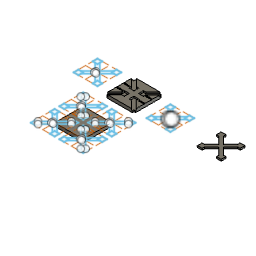
Bodenplatte_1 (Autodesk Fusion 360 design; units mm, degrees)
Autodesk Fusion 360 part; units mm, degrees
note: some values were not read from the file. Set by a fixed rule: which face or edge a step refers to.
(part 1 of 2)
sketch "Skizze1" plane through (0, 0, 0) normal (0, 1, 0) x (1, 0, 0)
  line L0 (-45, 40) -> (-45, -40)
  line L1 (-45, -40) -> (-40, -40)
  line L2 (-40, -40) -> (-40, -45)
  line L3 (-40, -45) -> (40, -45)
  line L4 (40, -45) -> (40, -40)
  line L5 (40, -40) -> (45, -40)
  line L6 (45, -40) -> (45, 40)
  line L7 (45, 40) -> (40, 40)
  line L8 (40, 40) -> (40, 45)
  line L9 (40, 45) -> (-40, 45)
  line L10 (-40, 45) -> (-40, 40)
  line L11 (-40, 40) -> (-45, 40)
  constraint vertical L0
  constraint perpendicular L0 L1
  constraint perpendicular L1 L2
  constraint perpendicular L2 L3
  constraint perpendicular L3 L4
  constraint perpendicular L4 L5
  constraint perpendicular L5 L6
  constraint perpendicular L6 L7
  constraint perpendicular L7 L8
  constraint perpendicular L8 L9
  constraint perpendicular L9 L10
  constraint perpendicular L0 L11
extrude "Extrusion1" add sketch "Skizze1" along normal blind 10 makes body 1
ref_plane "Arbeitsebene3" through (-45, 10, -40) normal (0, -1, 0) x (1, 0, 0)
sketch "Skizze5" plane through (0, 10, 0) normal (0, -1, 0) x (-1, 0, 0)
  line L0 (-7.5, -67.5) -> (-7.5, -82.5)
  line L1 (-22.5, -75) -> (-75, -22.5)
  line L2 (-75, -67.5) -> (-22.5, -15)
  line L3 (-67.5, -7.5) -> (-67.5, -22.5)
  line L4 (-22.5, -7.5) -> (-22.5, -22.5)
  line L5 (-7.5, -7.5) -> (-7.5, -82.5) construction
  line L6 (-15, -22.5) -> (-67.5, -75)
  line L7 (-67.5, -67.5) -> (-82.5, -67.5)
  line L8 (-7.5, -7.5) -> (-22.5, -7.5)
  line L9 (-22.5, -67.5) -> (-7.5, -67.5)
  line L10 (-7.5, -22.5) -> (-7.5, -7.5)
  line L11 (-7.5, -82.5) -> (-22.5, -82.5)
  line L12 (-22.5, -22.5) -> (-7.5, -22.5)
  line L13 (-45, -82.5) -> (-45, -7.5) construction
  line L14 (-22.5, -82.5) -> (-22.5, -67.5)
  line L15 (-67.5, -22.5) -> (-82.5, -22.5)
  line L16 (-82.5, -7.5) -> (-7.5, -7.5) construction
  line L17 (-82.5, -22.5) -> (-82.5, -7.5)
  line L18 (-7.5, -82.5) -> (-82.5, -82.5) construction
  line L19 (-67.5, -82.5) -> (-67.5, -67.5)
  line L20 (-82.5, -67.5) -> (-82.5, -82.5)
  line L21 (-82.5, -82.5) -> (-82.5, -7.5) construction
  line L22 (-82.5, -82.5) -> (-67.5, -82.5)
  line L23 (-82.5, -7.5) -> (-67.5, -7.5)
  line L24 (-15, -67.5) -> (-67.5, -15)
  line L25 (-7.5, -45) -> (-82.5, -45) construction
  line L26 (-7.4, -22.6) -> (-7.4, -7.4)
  line L27 (-7.4, -7.4) -> (-22.6, -7.4)
  line L28 (-22.6, -7.4) -> (-22.6, -22.6)
  line L29 (-22.6, -22.6) -> (-7.4, -22.6)
  line L30 (-75.0707, -67.4293) -> (-22.5707, -14.9293)
  line L31 (-14.9293, -22.5707) -> (-67.4293, -75.0707)
  point P0 (-40, -50)
  point P1 (-45, -50)
  point P2 (-40, -45)
  dimension "d20" = 75
  dimension "d21" = 75
  dimension "d22" = 0.1
  dimension "d23" = -0.1
  dimension "d24" = -0.1
  constraint horizontal L18
  constraint vertical L21
  constraint horizontal L16
  constraint vertical L5
  constraint horizontal L11
  constraint vertical L14
  constraint horizontal L9
  constraint vertical L0
  constraint horizontal L22
  constraint vertical L19
  constraint horizontal L7
  constraint vertical L20
  constraint horizontal L8
  constraint vertical L4
  constraint horizontal L12
  constraint vertical L10
  constraint horizontal L23
  constraint vertical L3
  constraint horizontal L15
  constraint vertical L17
  constraint midpoint L6.start L12
  constraint midpoint L6.end L19
  constraint midpoint L2.start L7
  constraint midpoint L2.end L4
  constraint midpoint L24.start L9
  constraint midpoint L24.end L3
  constraint midpoint L1.start L14
  constraint midpoint L1.end L15
  constraint midpoint L13.start L18
  constraint midpoint L13.end L16
  constraint midpoint L25.start L5
  constraint midpoint L25.end L21
  measures "d20" distance of L0.end L18.end
  measures "d21" distance of L5.start L0.end
extrude "Extrusion2" cut sketch "Skizze5" along normal blind 5 contours L1 L6 L24 L31 | L6 L24 L29 L31 | L2 L6 L24 L28 L29 | L1 L2 L6 L24 | L2 L4 L6 L8 L10 L12 L26 L27 L28 L29 | L2 L4 L6 L12 L28 L29 | L2 L24 L28 L30 | L1 L2 L24 L30 | L4 L8 L10 L12 bodies 1
ref_plane "Arbeitsebene4" through (-45, 10, -40) normal (0, -1, 0) x (1, 0, 0)
sketch "Skizze6" plane through (0, 10, 0) normal (0, -1, 0) x (-1, 0, 0)
  line L0 (-26.2733, -14.8317) -> (-41.3593, -14.8317) construction
  line L1 (-41.3593, -14.8317) -> (-41.3593, -8.56) construction
  line L2 (-41.3593, -8.56) -> (-26.2733, -8.56) construction
  line L3 (-26.2733, -8.56) -> (-26.2733, -14.8317) construction
  dimension "d27" = 4
  text T0 "0,1mm" font "Arial" height 4 align left top in box 15.086 x 6.2717 at (-26.2733, -14.8317) x (-1, 0) y (0, 1) spacing 1 kerned
extrude "Extrusion3" cut sketch "Skizze6" along normal blind 1 text T0 bodies 1
ref_plane "Arbeitsebene5" through (-45, 10, -40) normal (0, -1, 0) x (1, 0, 0)
sketch "Skizze7" plane through (0, 10, 0) normal (0, -1, 0) x (-1, 0, 0)
  line L0 (82.5, -67.5) -> (82.5, -82.5)
  line L1 (67.5, -75) -> (15, -22.5)
  line L2 (15, -67.5) -> (67.5, -15)
  line L3 (22.5, -7.5) -> (22.5, -22.5)
  line L4 (67.5, -7.5) -> (67.5, -22.5)
  line L5 (82.5, -7.5) -> (82.5, -82.5) construction
  line L6 (75, -22.5) -> (22.5, -75)
  line L7 (22.5, -67.5) -> (7.5, -67.5)
  line L8 (82.5, -7.5) -> (67.5, -7.5)
  line L9 (67.5, -67.5) -> (82.5, -67.5)
  line L10 (82.5, -22.5) -> (82.5, -7.5)
  line L11 (82.5, -82.5) -> (67.5, -82.5)
  line L12 (67.5, -22.5) -> (82.5, -22.5)
  line L13 (45, -82.5) -> (45, -7.5) construction
  line L14 (67.5, -82.5) -> (67.5, -67.5)
  line L15 (22.5, -22.5) -> (7.5, -22.5)
  line L16 (7.5, -7.5) -> (82.5, -7.5) construction
  line L17 (7.5, -22.5) -> (7.5, -7.5)
  line L18 (82.5, -82.5) -> (7.5, -82.5) construction
  line L19 (22.5, -82.5) -> (22.5, -67.5)
  line L20 (7.5, -67.5) -> (7.5, -82.5)
  line L21 (7.5, -82.5) -> (7.5, -7.5) construction
  line L22 (7.5, -82.5) -> (22.5, -82.5)
  line L23 (7.5, -7.5) -> (22.5, -7.5)
  line L24 (75, -67.5) -> (22.5, -15)
  line L25 (82.5, -45) -> (7.5, -45) construction
  line L26 (75.1061, -67.3939) -> (22.6061, -14.8939)
  line L27 (67.3939, -75.1061) -> (14.8939, -22.6061)
  line L28 (7.35, -7.35) -> (22.65, -7.35)
  line L29 (22.65, -7.35) -> (22.65, -22.65)
  line L30 (22.65, -22.65) -> (7.35, -22.65)
  line L31 (7.35, -22.65) -> (7.35, -7.35)
  point P0 (50, -50)
  point P1 (45, -50)
  point P2 (50, -45)
  dimension "d30" = 75
  dimension "d31" = 75
  dimension "d32" = 0.15
  dimension "d33" = -0.15
  dimension "d34" = -0.15
  constraint horizontal L18
  constraint vertical L21
  constraint horizontal L16
  constraint vertical L5
  constraint horizontal L11
  constraint vertical L14
  constraint horizontal L9
  constraint vertical L0
  constraint horizontal L22
  constraint vertical L19
  constraint horizontal L7
  constraint vertical L20
  constraint horizontal L8
  constraint vertical L4
  constraint horizontal L12
  constraint vertical L10
  constraint horizontal L23
  constraint vertical L3
  constraint horizontal L15
  constraint vertical L17
  constraint midpoint L6.start L12
  constraint midpoint L6.end L19
  constraint midpoint L2.start L7
  constraint midpoint L2.end L4
  constraint midpoint L24.start L9
  constraint midpoint L24.end L3
  constraint midpoint L1.start L14
  constraint midpoint L1.end L15
  constraint midpoint L13.start L18
  constraint midpoint L13.end L16
  constraint midpoint L25.start L5
  constraint midpoint L25.end L21
  measures "d30" distance of L0.end L18.end
  measures "d31" distance of L5.start L0.end
extrude "Extrusion4" cut sketch "Skizze7" along normal blind 5 contours L2 L6 L24 L26 | L1 L2 L6 L24 | L1 L2 L6 L27 | L2 L24 L26 L29 | L1 L2 L24 L29 L30 | L1 L2 L27 L30 | L1 L3 L15 L24 L29 L30 | L1 L3 L15 L17 L23 L24 L28 L29 L30 L31 | L3 L15 L17 L23 bodies 1
ref_plane "Arbeitsebene6" through (-45, 10, -40) normal (0, -1, 0) x (1, 0, 0)
sketch "Skizze8" plane through (0, 10, 0) normal (0, -1, 0) x (-1, 0, 0)
  line L0 (43.5802, -15.8742) -> (43.5801, -15.8742) construction
  line L1 (43.5801, -15.8742) -> (43.7283, -9.6192) construction
  line L2 (43.7283, -9.6192) -> (43.7284, -9.6192) construction
  line L3 (43.7284, -9.6192) -> (43.5802, -15.8742) construction
  line L4 (82.5, 22.5) -> (82.5, 7.5)
  line L5 (67.5, 15) -> (15, 67.5)
  line L6 (15, 22.5) -> (67.5, 75)
  line L7 (22.5, 82.5) -> (22.5, 67.5)
  line L8 (67.5, 82.5) -> (67.5, 67.5)
  line L9 (82.5, 82.5) -> (82.5, 7.5) construction
  line L10 (75, 67.5) -> (22.5, 15)
  line L11 (22.5, 22.5) -> (7.5, 22.5)
  line L12 (82.5, 82.5) -> (67.5, 82.5)
  line L13 (67.5, 22.5) -> (82.5, 22.5)
  line L14 (82.5, 67.5) -> (82.5, 82.5)
  line L15 (82.5, 7.5) -> (67.5, 7.5)
  line L16 (67.5, 67.5) -> (82.5, 67.5)
  line L17 (45, 7.5) -> (45, 82.5) construction
  line L18 (67.5, 7.5) -> (67.5, 22.5)
  line L19 (22.5, 67.5) -> (7.5, 67.5)
  line L20 (7.5, 82.5) -> (82.5, 82.5) construction
  line L21 (7.5, 67.5) -> (7.5, 82.5)
  line L22 (82.5, 7.5) -> (7.5, 7.5) construction
  line L23 (22.5, 7.5) -> (22.5, 22.5)
  line L24 (7.5, 22.5) -> (7.5, 7.5)
  line L25 (7.5, 7.5) -> (7.5, 82.5) construction
  line L26 (7.5, 7.5) -> (22.5, 7.5)
  line L27 (7.5, 82.5) -> (22.5, 82.5)
  line L28 (75, 22.5) -> (22.5, 75)
  line L29 (82.5, 45) -> (7.5, 45) construction
  line L30 (14.8586, 22.6414) -> (67.3586, 75.1414)
  line L31 (75.1414, 67.3586) -> (22.6414, 14.8586)
  line L32 (22.7, 22.7) -> (7.3, 22.7)
  line L33 (7.3, 22.7) -> (7.3, 7.3)
  line L34 (7.3, 7.3) -> (22.7, 7.3)
  line L35 (22.7, 7.3) -> (22.7, 22.7)
  line L36 (-7.5, 22.5) -> (-7.5, 7.5)
  line L37 (-22.5, 15) -> (-75, 67.5)
  line L38 (-75, 22.5) -> (-22.5, 75)
  line L39 (-67.5, 82.5) -> (-67.5, 67.5)
  line L40 (-22.5, 82.5) -> (-22.5, 67.5)
  line L41 (-7.5, 82.5) -> (-7.5, 7.5) construction
  line L42 (-15, 67.5) -> (-67.5, 15)
  line L43 (-67.5, 22.5) -> (-82.5, 22.5)
  line L44 (-7.5, 82.5) -> (-22.5, 82.5)
  line L45 (-22.5, 22.5) -> (-7.5, 22.5)
  line L46 (-7.5, 67.5) -> (-7.5, 82.5)
  line L47 (-7.5, 7.5) -> (-22.5, 7.5)
  line L48 (-22.5, 67.5) -> (-7.5, 67.5)
  line L49 (-45, 7.5) -> (-45, 82.5) construction
  line L50 (-22.5, 7.5) -> (-22.5, 22.5)
  line L51 (-67.5, 67.5) -> (-82.5, 67.5)
  line L52 (-82.5, 82.5) -> (-7.5, 82.5) construction
  line L53 (-82.5, 67.5) -> (-82.5, 82.5)
  line L54 (-7.5, 7.5) -> (-82.5, 7.5) construction
  line L55 (-67.5, 7.5) -> (-67.5, 22.5)
  line L56 (-82.5, 22.5) -> (-82.5, 7.5)
  line L57 (-82.5, 7.5) -> (-82.5, 82.5) construction
  line L58 (-82.5, 7.5) -> (-67.5, 7.5)
  line L59 (-82.5, 82.5) -> (-67.5, 82.5)
  line L60 (-15, 22.5) -> (-67.5, 75)
  line L61 (-7.5, 45) -> (-82.5, 45) construction
  line L62 (-22.6768, 14.8232) -> (-75.1768, 67.3232)
  line L63 (-14.8232, 22.6768) -> (-67.3232, 75.1768)
  line L64 (-7.25, 7.25) -> (-22.75, 7.25)
  line L65 (-22.75, 7.25) -> (-22.75, 22.75)
  line L66 (-22.75, 22.75) -> (-7.25, 22.75)
  line L67 (-7.25, 22.75) -> (-7.25, 7.25)
  line L68 (43.7513, 9) -> (26, 9) construction
  line L69 (26, 9) -> (26, 17.5106) construction
  line L70 (26, 17.5106) -> (43.7513, 17.5106) construction
  line L71 (43.7513, 17.5106) -> (43.7513, 9) construction
  line L72 (-24.3671, 8.4428) -> (-42.7802, 8.4428) construction
  line L73 (-42.7802, 8.4428) -> (-42.7802, 14.5497) construction
  line L74 (-42.7802, 14.5497) -> (-24.3671, 14.5497) construction
  line L75 (-24.3671, 14.5497) -> (-24.3671, 8.4428) construction
  point P0 (50, 40)
  point P1 (45, 40)
  point P2 (50, 45)
  point P3 (-40, 40)
  point P4 (-45, 40)
  point P5 (-40, 45)
  dimension "d37" = 4
  dimension "d38" = 75
  dimension "d39" = 75
  dimension "d40" = -0.2
  dimension "d41" = -0.2
  dimension "d42" = 0.2
  dimension "d43" = 75
  dimension "d44" = 75
  dimension "d45" = -0.25
  dimension "d46" = 0.25
  dimension "d47" = -0.25
  dimension "d48" = 4
  dimension "d49" = 4
  constraint horizontal L22
  constraint vertical L25
  constraint horizontal L20
  constraint vertical L9
  constraint horizontal L15
  constraint vertical L18
  constraint horizontal L13
  constraint vertical L4
  constraint horizontal L26
  constraint vertical L23
  constraint horizontal L11
  constraint vertical L24
  constraint horizontal L12
  constraint vertical L8
  constraint horizontal L16
  constraint vertical L14
  constraint horizontal L27
  constraint vertical L7
  constraint horizontal L19
  constraint vertical L21
  constraint midpoint L10.start L16
  constraint midpoint L10.end L23
  constraint midpoint L6.start L11
  constraint midpoint L6.end L8
  constraint midpoint L28.start L13
  constraint midpoint L28.end L7
  constraint midpoint L5.start L18
  constraint midpoint L5.end L19
  constraint midpoint L17.start L22
  constraint midpoint L17.end L20
  constraint midpoint L29.start L9
  constraint midpoint L29.end L25
  constraint horizontal L54
  constraint vertical L57
  constraint horizontal L52
  constraint vertical L41
  constraint horizontal L47
  constraint vertical L50
  constraint horizontal L45
  constraint vertical L36
  constraint horizontal L58
  constraint vertical L55
  constraint horizontal L43
  constraint vertical L56
  constraint horizontal L44
  constraint vertical L40
  constraint horizontal L48
  constraint vertical L46
  constraint horizontal L59
  constraint vertical L39
  constraint horizontal L51
  constraint vertical L53
  constraint midpoint L42.start L48
  constraint midpoint L42.end L55
  constraint midpoint L38.start L43
  constraint midpoint L38.end L40
  constraint midpoint L60.start L45
  constraint midpoint L60.end L39
  constraint midpoint L37.start L50
  constraint midpoint L37.end L51
  constraint midpoint L49.start L54
  constraint midpoint L49.end L52
  constraint midpoint L61.start L41
  constraint midpoint L61.end L57
  measures "d38" distance of L4.end L22.end
  measures "d39" distance of L9.start L4.end
  measures "d43" distance of L36.end L54.end
  measures "d44" distance of L41.start L36.end
sketch "Skizze9" plane through (0, 0, 0) normal (0, 0, 1) x (1, 0, 0)
extrude "Extrusion5" cut sketch "Skizze8" along normal blind 5 contours L5 L10 L28 L31 | L5 L6 L10 L28 | L5 L10 L31 L35 | L5 L6 L10 L32 L35 | L5 L6 L28 L30 | L6 L10 L11 L23 L24 L26 L32 L33 L34 L35 | L5 L6 L30 L32 | L6 L10 L11 L23 L32 L35 | L11 L23 L24 L26 | L36 L37 L45 L47 L50 L60 L64 L65 L66 L67 | L36 L45 L47 L50 | L37 L45 L50 L60 L65 L66 | L37 L42 L60 L65 L66 | L42 L60 L63 L66 | L38 L42 L60 L63 | L37 L38 L42 L60 | L37 L42 L62 L65 | L37 L38 L42 L62 bodies 1
ref_plane "Arbeitsebene7" through (-45, 10, -37.2172) normal (0, -1, 0) x (1, 0, 0)
sketch "Skizze10" plane through (0, 10, 0) normal (0, -1, 0) x (-1, 0, 0)
  line L0 (44, -14) -> (25, -14) construction
  line L1 (25, -14) -> (25, -7) construction
  line L2 (25, -7) -> (44, -7) construction
  line L3 (44, -7) -> (44, -14) construction
  line L4 (43, 8.2933) -> (24.4104, 8.2933) construction
  line L5 (24.4104, 8.2933) -> (24.4104, 15) construction
  line L6 (24.4104, 15) -> (43, 15) construction
  line L7 (43, 15) -> (43, 8.2933) construction
  line L8 (-24, 9) -> (-42, 9) construction
  line L9 (-42, 9) -> (-42, 15) construction
  line L10 (-42, 15) -> (-24, 15) construction
  line L11 (-24, 15) -> (-24, 9) construction
  dimension "d52" = 4
  dimension "d53" = 4
  dimension "d54" = 4
  text T0 "0,15mm" font "Arial" height 4 align left top in box 19 x 7 at (44, -14) x (-1, 0) y (0, 1) spacing 1 kerned
  text T1 "0,2mm" font "Arial" height 4 align left top in box 18.5896 x 6.7067 at (43, 8.2933) x (-1, 0) y (0, 1) spacing 1 kerned
  text T2 "0,25mm" font "Arial" height 4 align left top in box 18 x 6 at (-24, 9) x (-1, 0) y (0, 1) spacing 1 kerned
extrude "Extrusion6" cut sketch "Skizze10" along normal blind 1 text T2 T1 T0 bodies 1
sketch "Skizze11" plane through (0, 0, 0) normal (0, 0, 1) x (1, 0, 0)
sketch "Skizze12" plane through (0, 0, 0) normal (0, 1, 0) x (1, 0, 0)
  line L0 (152.5, -22.5) -> (152.5, -37.5)
  line L1 (137.5, -30) -> (85, 22.5)
  line L2 (85, -22.5) -> (137.5, 30)
  line L3 (92.5, 37.5) -> (92.5, 22.5)
  line L4 (137.5, 37.5) -> (137.5, 22.5)
  line L5 (152.5, 37.5) -> (152.5, -37.5) construction
  line L6 (145, 22.5) -> (92.5, -30)
  line L7 (92.5, -22.5) -> (77.5, -22.5)
  line L8 (152.5, 37.5) -> (137.5, 37.5)
  line L9 (137.5, -22.5) -> (152.5, -22.5)
  line L10 (152.5, 22.5) -> (152.5, 37.5)
  line L11 (152.5, -37.5) -> (137.5, -37.5)
  line L12 (137.5, 22.5) -> (152.5, 22.5)
  line L13 (115, -37.5) -> (115, 37.5) construction
  line L14 (137.5, -37.5) -> (137.5, -22.5)
  line L15 (92.5, 22.5) -> (77.5, 22.5)
  line L16 (77.5, 37.5) -> (152.5, 37.5) construction
  line L17 (77.5, 22.5) -> (77.5, 37.5)
  line L18 (152.5, -37.5) -> (77.5, -37.5) construction
  line L19 (92.5, -37.5) -> (92.5, -22.5)
  line L20 (77.5, -22.5) -> (77.5, -37.5)
  line L21 (77.5, -37.5) -> (77.5, 37.5) construction
  line L22 (77.5, -37.5) -> (92.5, -37.5)
  line L23 (77.5, 37.5) -> (92.5, 37.5)
  line L24 (145, -22.5) -> (92.5, 30)
  line L25 (152.5, 0) -> (77.5, 0) construction
  point P0 (120, -5)
  point P1 (115, -5)
  point P2 (120, 0)
  dimension "d57" = 75
  dimension "d58" = 75
  constraint horizontal L18
  constraint vertical L21
  constraint horizontal L16
  constraint vertical L5
  constraint horizontal L11
  constraint vertical L14
  constraint horizontal L9
  constraint vertical L0
  constraint horizontal L22
  constraint vertical L19
  constraint horizontal L7
  constraint vertical L20
  constraint horizontal L8
  constraint vertical L4
  constraint horizontal L12
  constraint vertical L10
  constraint horizontal L23
  constraint vertical L3
  constraint horizontal L15
  constraint vertical L17
  constraint midpoint L6.start L12
  constraint midpoint L6.end L19
  constraint midpoint L2.start L7
  constraint midpoint L2.end L4
  constraint midpoint L24.start L9
  constraint midpoint L24.end L3
  constraint midpoint L1.start L14
  constraint midpoint L1.end L15
  constraint midpoint L13.start L18
  constraint midpoint L13.end L16
  constraint midpoint L25.start L5
  constraint midpoint L25.end L21
  measures "d57" distance of L0.end L18.end
  measures "d58" distance of L5.start L0.end
extrude "Extrusion7" add sketch "Skizze12" along normal blind 5 separate body makes body 2
copy_body "Körper kopieren/einfügen1" bodies 2 makes body 3
move_body "Verschieben2" bodies 3 to x (1, 0, 0) y (0, 1, 0) z (0, 0, 1) at (160, 0, 0)
copy_body "Körper kopieren/einfügen2" bodies 1 makes body 4
move_body "Verschieben3" bodies 4 to x (1, 0, 0) y (0, 1, 0) z (0, 0, 1) at (0, 0, 160)
extrude "Extrusion8" add 4 faces at (25.8821, 5, 134.1179) (-25.8724, 5, 134.1276) (-25.8626, 5, 185.8626) (25.8529, 5, 185.8529) along direction (0, 1, 0) blind 5 on bodies 4 bodies 4
delete_face "Fläche löschen1" 236 faces at (-29.9479, 9.5, 147.3795) (-40.0682, 9.3333, 170.6271) (-24.5694, 9.6667, 171) (-30.9386, 9.6667, 171) (-31.697, 9.5, 168.4677) (-34.6562, 9.6667, 146.2378) (-40.5885, 9.5, 148.2966) (-42.7174, 9.5, 148.4385) (-41.5585, 9.5, 149.059) (-41.8758, 9.5, 149.0506) (-42.4956, 9.5, 147.3048) (-42.1855, 9.5, 148.4319) (-41.206, 9.5, 148.4309) (-41.0614, 9.5, 148.1749) (-40.8959, 9.5, 146.7492) (-42.3137, 9.5, 145.8483) (-42.6525, 9, 147.3777) (-26.6771, 9.6667, 149) (-35.0941, 9.6667, 167.0546) (-30.162, 9.5, 168.4713) (-31.1692, 9.3333, 147.6739) (-39.0716, 9.5, 149.0942) (-39.4515, 9.5, 149.7541) (-39.5694, 9.3333, 149.7212) (-26.1201, 9.6667, 169.8777) (-34.0396, 9.5, 170.7219) (-41.5885, 9.5, 170.2966) (-43.7174, 9.5, 170.4385) (-30.2769, 9, 147.533) (-42.5585, 9.5, 171.059) (-37.1921, 9.5, 147.3665) (-42.8758, 9.5, 171.0506) (-37.1319, 9.5, 145.3985) (-43.4956, 9.5, 169.3048) (-43.1855, 9.5, 170.4319) (-37.7964, 9.5, 146.0767) (-29.0614, 9.3333, 169.6739) (-33.3766, 9.5, 147.0199) (-29.2242, 9.6667, 171) (-34.1096, 9.5, 169.5582) (-33.3738, 9.3333, 148.3724) (-26.075, 9.5, 168.3987) (-40.0716, 9.5, 171.0942) (-35.4361, 9.6667, 167.8822) (-32.8376, 9.5, 146.3987) (-24.895, 9.3333, 170.3915) (-35.4598, 9.5, 168.5269) (-40.4515, 9.5, 171.7541) (-32.9926, 9.5, 146.4694) (-24.8954, 9.5, 169.0897) (-27.0032, 9.5, 147.0897) (-33.6782, 9.5, 146.0414) (-40.5694, 9.3333, 171.7212) (-34.6573, 9.5, 168.3643) (-25.0779, 9.5, 168.5699) (-27.1856, 9.5, 146.5699) (-33.5948, 9.5, 169.4652) (-40.442, 9.6667, 171) (-31.266, 9.3333, 170.3724) (-25.357, 9.5, 168.4657) (-27.4647, 9.5, 146.4657) (-29.8401, 9.5, 146.8259) (-30.1132, 9.6667, 149) (-42.206, 9.5, 170.4309) (-32.1196, 9.5, 146.4657) (-31.8405, 9.5, 146.5699) (-26.5206, 9.5, 146.8624) (-35.8372, 9.3333, 169.1492) (-31.658, 9.5, 147.0897) (-31.6576, 9.3333, 148.3915) (-26.5143, 9.3333, 147.6739) (-36.0155, 9.6667, 168.4243) (-31.332, 9.6667, 149) (-30.0118, 9.5, 168.4657) (-29.5498, 9.3333, 170.3915) (-33.0464, 9.6667, 149) (-34.8357, 9.5, 168.7917) (-29.5503, 9.5, 169.0897) (-41.8959, 9.5, 168.7492) (-43.3137, 9.5, 167.8483) (-34.3645, 9.5, 146.2132) (-40.6126, 9.5, 171.5561) (-31.9326, 9.5, 146.045) (-33.5936, 9.5, 169.8169) (-40.3483, 9, 170.6271) (-25.5071, 9.5, 168.4713) (-36.2033, 9.5, 170.11) (-27.6149, 9.5, 146.4713) (-38.0896, 9.5, 148.2126) (-37.5053, 9.5, 147.6264) (-42.2066, 9.5, 167.6217) (-39.4411, 9.6667, 148.4407) (-42.4342, 10, 168.7024) (-39.0682, 9.3333, 148.6271) (-43.1684, 9.5, 167.5944) (-40.3533, 9.5, 171.074) (-33.8048, 9.5, 146.4677) (-29.0676, 9.5, 168.8624) (-37.1865, 9.5, 144.9942) (-37.2938, 9, 148.8427) (-37.0677, 9.5, 147.8608) (-37.5523, 9.5, 148.3053) (-43.6525, 9, 169.3777) (-39.6276, 9.3333, 148.8136) (-28.0055, 9.6667, 171) (-32.495, 9.5, 169.3795) (-42.8323, 9.5, 166.9929) (-38.4011, 9.5, 148.9416) (-28.1692, 9, 169.533) (-32.4966, 9.6667, 169.9977) (-42.5937, 9.5, 166.9888) (-25.17, 9.5, 168.045) (-31.1754, 9.5, 146.8624) (-30.77, 9.5, 169.1837) (-27.0027, 9.3333, 148.3915) (-34.3001, 9.6667, 167.5239) (-32.2567, 9.5, 168.2132) (-37.4898, 9.3333, 168.3224) (-29.0234, 9.5, 146.0414) (-27.6018, 9.5, 168.2132) (-36.2783, 9.5, 145.9902) (-28.3377, 9.5, 146.4694) (-27.1075, 9.5, 168.0423) (-36.4323, 9.5, 146.5757) (-31.7624, 9.5, 168.0423) (-37.6535, 9, 168.618) (-35.7585, 9.6667, 148.6853) (-34.4331, 9.5, 170.4737) (-31.5705, 9.5, 168.0414) (-34.6044, 9.6667, 147.9977) (-34.1102, 9.5, 169.8244) (-30.8848, 9.5, 168.4694) (-34.6028, 9.5, 147.3795) (-38.1506, 9.5, 167.4315) (-26.9156, 9.5, 168.0414) (-30.7298, 9.5, 168.3987) (-28.1828, 9.5, 146.3987) (-34.9318, 9, 147.533) (-26.23, 9.5, 168.4694) (-37.7008, 9.6667, 166.9836) (-34.7681, 9.6667, 149) (-33.8702, 9.5, 146.0423) (-31.2689, 9.5, 169.0199) (-41.786, 9.5, 167.4112) (-29.15, 9.5, 146.4677) (-33.7681, 9.3333, 167.211) (-41.2066, 9.5, 145.6217) (-41.4342, 10, 146.7024) (-28.2229, 9.5, 147.1837) (-26.2838, 9.6667, 171) (-43.9961, 9.5, 168.8128) (-35.0955, 9.6667, 148.0341) (-28.2278, 9.6667, 147.8777) (-32.3872, 9.5, 168.8259) (-26.6112, 9.3333, 170.3724) (-32.6603, 9.6667, 171) (-26.614, 9.5, 169.0199) (-43.8014, 9.5, 167.7526) (-28.3915, 9.6667, 149) (-35.1168, 9.5, 171.0563) (-27.0422, 9.5, 168.4677) (-28.719, 9.3333, 148.3724) (-32.824, 9, 169.533) (-27.1918, 9.5, 168.4675) (-27.7324, 9.5, 168.8259) (-36.6398, 9.6667, 149) (-33.9544, 9.5, 146.4675) (-29.8248, 9.5, 168.045) (-37.9732, 9.6667, 146.1751) (-42.0614, 9.5, 170.1749) (-28.7218, 9.5, 147.0199) (-30.7749, 9.6667, 169.8777) (-34.495, 9.5, 146.8259) (-38.2827, 9.5, 145.968) (-32.8827, 9.6667, 147.8777) (-35.0313, 9.5, 168.7864) (-32.8778, 9.5, 147.1837) (-40.6276, 9.3333, 170.8136) (-24.4128, 9.5, 168.8624) (-35.4429, 9.5, 168.9279) (-27.2778, 9.5, 146.045) (-32.2698, 9.5, 146.4713) (-40.4411, 9.6667, 170.4407) (-24.4065, 9.3333, 169.6739) (-29.7327, 9.5, 168.5699) (-42.1684, 9.5, 145.5944) (-36.06, 9.6667, 169.9377) (-39.442, 9.6667, 149) (-39.3483, 9, 148.6271) (-39.6126, 9.5, 149.5561) (-39.3533, 9.5, 149.074) (-42.9961, 9.5, 146.8128) (-42.8014, 9.5, 145.7526) (-41.8323, 9.5, 144.9929) (-41.5937, 9.5, 144.9888) (-40.786, 9.5, 145.4112) (-40.5133, 9.5, 145.9722) (-40.3937, 9.5, 146.8488) (-40.3955, 9.5, 147.2404) (-26.1151, 9.5, 169.1837) (-34.9632, 9, 167.211) (-41.5133, 9.5, 167.9722) (-41.3937, 9.5, 168.8488) (-29.2996, 9.5, 146.4675) (-41.3955, 9.5, 169.2404) (-31.8467, 9.5, 168.4675) (-34.9491, 9.6667, 146.1023) (-27.8401, 9.5, 169.3795) (-38.3577, 9.5, 168.1546) (-28.1864, 9.6667, 168.1023) (-30.0014, 9.6667, 146.2378) (-35.693, 9.5, 170.0227) (-32.8413, 9.6667, 168.1023) (-38.5362, 9.5, 168.26) (-32.9877, 9.6667, 170.0341) (-37.6535, 9.6667, 171) (-37.0664, 9.6667, 148.528) (-35.7793, 9.5, 145.9441) (-29.2153, 9.5, 146.0423) (-36.8336, 9.5, 144.9953) (-38.8318, 9.5, 167.9204) (-35.0407, 9.5, 170.656) (-27.8936, 9.6667, 168.2378) (-36.1197, 9.5, 146.9734) (-30.2942, 9.6667, 146.1023) (-35.834, 9.5, 146.4889) (-29.9495, 9.6667, 147.9977) (-27.8417, 9.6667, 169.9977) (-36.7918, 9.5, 147.6278) (-30.4407, 9.6667, 148.0341) (-29.7096, 9.5, 146.2132) (-37.9809, 9.3333, 169.9568) (-28.3329, 9.6667, 170.0341) (-38.9632, 9.6667, 168.3042) (-32.5484, 9.6667, 168.2378) (-36.9172, 9.5, 145.3982) on bodies 4
extrude "Extrusion9" add 6 faces at (24.3475, 9, 147.3777) (27.6517, 9, 148.6271) (29.7062, 9, 148.8427) (33.0368, 9, 145.211) (35.176, 9, 147.533) (39.8308, 9, 147.533) along direction (0, 1, 0) blind 1 on bodies 4 bodies 4
extrude "Extrusion10" add 5 faces at (26.6208, 9, 170.9377) (29.925, 9, 172.1871) (32.6198, 9, 170.178) (34.3415, 9, 171.093) (38.9964, 9, 171.093) along direction (0, 1, 0) blind 1 on bodies 4 bodies 4
ref_plane "Arbeitsebene8" through (-45, 10, 120) normal (0, -1, 0) x (1, 0, 0)
sketch "Skizze13" plane through (0, 10, 0) normal (0, -1, 0) x (-1, 0, 0)
  line L0 (77.5, -37.5) -> (92.5, -37.5)
  line L1 (152.5, -37.5) -> (77.5, -37.5) construction
  line L2 (77.5, 22.5) -> (77.5, 37.5)
  line L3 (137.5, -22.5) -> (152.5, -22.5)
  line L4 (152.5, -22.5) -> (152.5, -37.5)
  line L5 (152.5, 0) -> (77.5, 0) construction
  line L6 (145, -22.5) -> (92.5, 30)
  line L7 (92.5, -37.5) -> (92.5, -22.5)
  line L8 (137.5, 37.5) -> (137.5, 22.5)
  line L9 (137.5, 22.5) -> (152.5, 22.5)
  line L10 (77.5, 37.5) -> (152.5, 37.5) construction
  line L11 (152.5, 22.5) -> (152.5, 37.5)
  line L12 (115, -37.5) -> (115, 37.5) construction
  line L13 (77.5, -37.5) -> (77.5, 37.5) construction
  line L14 (145, 22.5) -> (92.5, -30)
  line L15 (137.5, -30) -> (85, 22.5)
  line L16 (85, -22.5) -> (137.5, 30)
  line L17 (152.5, 37.5) -> (152.5, -37.5) construction
  line L18 (152.5, 37.5) -> (137.5, 37.5)
  line L19 (92.5, 22.5) -> (77.5, 22.5)
  line L20 (77.5, -22.5) -> (77.5, -37.5)
  line L21 (152.5, -37.5) -> (137.5, -37.5)
  line L22 (92.5, -22.5) -> (77.5, -22.5)
  line L23 (77.5, 37.5) -> (92.5, 37.5)
  line L24 (92.5, 37.5) -> (92.5, 22.5)
  line L25 (137.5, -37.5) -> (137.5, -22.5)
  line L26 (-82.5, -242.5) -> (-67.5, -242.5)
  line L27 (-7.5, -242.5) -> (-82.5, -242.5) construction
  line L28 (-82.5, -182.5) -> (-82.5, -167.5)
  line L29 (-22.5, -227.5) -> (-7.5, -227.5)
  line L30 (-7.5, -227.5) -> (-7.5, -242.5)
  line L31 (-7.5, -205) -> (-82.5, -205) construction
  line L32 (-15, -227.5) -> (-67.5, -175)
  line L33 (-67.5, -242.5) -> (-67.5, -227.5)
  line L34 (-22.5, -167.5) -> (-22.5, -182.5)
  line L35 (-22.5, -182.5) -> (-7.5, -182.5)
  line L36 (-82.5, -167.5) -> (-7.5, -167.5) construction
  line L37 (-7.5, -182.5) -> (-7.5, -167.5)
  line L38 (-45, -242.5) -> (-45, -167.5) construction
  line L39 (-82.5, -242.5) -> (-82.5, -167.5) construction
  line L40 (-15, -182.5) -> (-67.5, -235)
  line L41 (-22.5, -235) -> (-75, -182.5)
  line L42 (-75, -227.5) -> (-22.5, -175)
  line L43 (-7.5, -167.5) -> (-7.5, -242.5) construction
  line L44 (-7.5, -167.5) -> (-22.5, -167.5)
  line L45 (-67.5, -182.5) -> (-82.5, -182.5)
  line L46 (-82.5, -227.5) -> (-82.5, -242.5)
  line L47 (-7.5, -242.5) -> (-22.5, -242.5)
  line L48 (-67.5, -227.5) -> (-82.5, -227.5)
  line L49 (-82.5, -167.5) -> (-67.5, -167.5)
  line L50 (-67.5, -167.5) -> (-67.5, -182.5)
  line L51 (-22.5, -242.5) -> (-22.5, -227.5)
  line L52 (7.5, -242.5) -> (22.5, -242.5)
  line L53 (82.5, -242.5) -> (7.5, -242.5) construction
  line L54 (7.5, -182.5) -> (7.5, -167.5)
  line L55 (67.5, -227.5) -> (82.5, -227.5)
  line L56 (82.5, -227.5) -> (82.5, -242.5)
  line L57 (82.5, -205) -> (7.5, -205) construction
  line L58 (75, -227.5) -> (22.5, -175)
  line L59 (22.5, -242.5) -> (22.5, -227.5)
  line L60 (67.5, -167.5) -> (67.5, -182.5)
  line L61 (67.5, -182.5) -> (82.5, -182.5)
  line L62 (7.5, -167.5) -> (82.5, -167.5) construction
  line L63 (82.5, -182.5) -> (82.5, -167.5)
  line L64 (45, -242.5) -> (45, -167.5) construction
  line L65 (7.5, -242.5) -> (7.5, -167.5) construction
  line L66 (75, -182.5) -> (22.5, -235)
  line L67 (67.5, -235) -> (15, -182.5)
  line L68 (15, -227.5) -> (67.5, -175)
  line L69 (82.5, -167.5) -> (82.5, -242.5) construction
  line L70 (82.5, -167.5) -> (67.5, -167.5)
  line L71 (22.5, -182.5) -> (7.5, -182.5)
  line L72 (7.5, -227.5) -> (7.5, -242.5)
  line L73 (82.5, -242.5) -> (67.5, -242.5)
  line L74 (22.5, -227.5) -> (7.5, -227.5)
  line L75 (7.5, -167.5) -> (22.5, -167.5)
  line L76 (22.5, -167.5) -> (22.5, -182.5)
  line L77 (67.5, -242.5) -> (67.5, -227.5)
  line L78 (-82.5, -152.5) -> (-67.5, -152.5)
  line L79 (-7.5, -152.5) -> (-82.5, -152.5) construction
  line L80 (-82.5, -92.5) -> (-82.5, -77.5)
  line L81 (-22.5, -137.5) -> (-7.5, -137.5)
  line L82 (-7.5, -137.5) -> (-7.5, -152.5)
  line L83 (-7.5, -115) -> (-82.5, -115) construction
  line L84 (-15, -137.5) -> (-67.5, -85)
  line L85 (-67.5, -152.5) -> (-67.5, -137.5)
  line L86 (-22.5, -77.5) -> (-22.5, -92.5)
  line L87 (-22.5, -92.5) -> (-7.5, -92.5)
  line L88 (-82.5, -77.5) -> (-7.5, -77.5) construction
  line L89 (-7.5, -92.5) -> (-7.5, -77.5)
  line L90 (-45, -152.5) -> (-45, -77.5) construction
  line L91 (-82.5, -152.5) -> (-82.5, -77.5) construction
  line L92 (-15, -92.5) -> (-67.5, -145)
  line L93 (-22.5, -145) -> (-75, -92.5)
  line L94 (-75, -137.5) -> (-22.5, -85)
  line L95 (-7.5, -77.5) -> (-7.5, -152.5) construction
  line L96 (-7.5, -77.5) -> (-22.5, -77.5)
  line L97 (-67.5, -92.5) -> (-82.5, -92.5)
  line L98 (-82.5, -137.5) -> (-82.5, -152.5)
  line L99 (-7.5, -152.5) -> (-22.5, -152.5)
  line L100 (-67.5, -137.5) -> (-82.5, -137.5)
  line L101 (-82.5, -77.5) -> (-67.5, -77.5)
  line L102 (-67.5, -77.5) -> (-67.5, -92.5)
  line L103 (-22.5, -152.5) -> (-22.5, -137.5)
  line L104 (7.5, -152.5) -> (22.5, -152.5)
  line L105 (82.5, -152.5) -> (7.5, -152.5) construction
  line L106 (7.5, -92.5) -> (7.5, -77.5)
  line L107 (67.5, -137.5) -> (82.5, -137.5)
  line L108 (82.5, -137.5) -> (82.5, -152.5)
  line L109 (82.5, -115) -> (7.5, -115) construction
  line L110 (75, -137.5) -> (22.5, -85)
  line L111 (22.5, -152.5) -> (22.5, -137.5)
  line L112 (67.5, -77.5) -> (67.5, -92.5)
  line L113 (67.5, -92.5) -> (82.5, -92.5)
  line L114 (7.5, -77.5) -> (82.5, -77.5) construction
  line L115 (82.5, -92.5) -> (82.5, -77.5)
  line L116 (45, -152.5) -> (45, -77.5) construction
  line L117 (7.5, -152.5) -> (7.5, -77.5) construction
  line L118 (75, -92.5) -> (22.5, -145)
  line L119 (67.5, -145) -> (15, -92.5)
  line L120 (15, -137.5) -> (67.5, -85)
  line L121 (82.5, -77.5) -> (82.5, -152.5) construction
  line L122 (82.5, -77.5) -> (67.5, -77.5)
  line L123 (22.5, -92.5) -> (7.5, -92.5)
  line L124 (7.5, -137.5) -> (7.5, -152.5)
  line L125 (82.5, -152.5) -> (67.5, -152.5)
  line L126 (22.5, -137.5) -> (7.5, -137.5)
  line L127 (7.5, -77.5) -> (22.5, -77.5)
  line L128 (22.5, -77.5) -> (22.5, -92.5)
  line L129 (67.5, -152.5) -> (67.5, -137.5)
  line L130 (-75.0707, -227.4293) -> (-22.5707, -174.9293) construction
  line L131 (-14.9293, -182.5707) -> (-67.4293, -235.0707) construction
  line L132 (-7.4, -182.6) -> (-7.4, -167.4) construction
  line L133 (-7.4, -167.4) -> (-22.6, -167.4) construction
  line L134 (-22.6, -167.4) -> (-22.6, -182.6) construction
  line L135 (-22.6, -182.6) -> (-7.4, -182.6) construction
  line L136 (-25.0826, -175) -> (-40, -175) construction
  line L137 (-40, -175) -> (-40, -167.5) construction
  line L138 (-40, -167.5) -> (-25.0826, -167.5) construction
  line L139 (-25.0826, -167.5) -> (-25.0826, -175) construction
  line L140 (75.0636, -227.4364) -> (22.5636, -174.9364) construction
  line L141 (67.4364, -235.0636) -> (14.9364, -182.5636) construction
  line L142 (7.41, -167.41) -> (22.59, -167.41) construction
  line L143 (22.59, -167.41) -> (22.59, -182.59) construction
  line L144 (22.59, -182.59) -> (7.41, -182.59) construction
  line L145 (7.41, -182.59) -> (7.41, -167.41) construction
  line L146 (39.9906, -175) -> (25, -175) construction
  line L147 (25, -175) -> (25, -167.5) construction
  line L148 (25, -167.5) -> (39.9906, -167.5) construction
  line L149 (39.9906, -167.5) -> (39.9906, -175) construction
  line L150 (14.9434, -137.4434) -> (67.4434, -84.9434) construction
  line L151 (75.0566, -92.5566) -> (22.5566, -145.0566) construction
  line L152 (7.42, -152.58) -> (22.58, -152.58) construction
  line L153 (22.58, -152.58) -> (22.58, -137.42) construction
  line L154 (22.58, -137.42) -> (7.42, -137.42) construction
  line L155 (7.42, -137.42) -> (7.42, -152.58) construction
  line L156 (40, -152.5) -> (24.7054, -152.5) construction
  line L157 (24.7054, -152.5) -> (24.7054, -145) construction
  line L158 (24.7054, -145) -> (40, -145) construction
  line L159 (40, -145) -> (40, -152.5) construction
  line L160 (-14.9505, -137.4505) -> (-67.4505, -84.9505) construction
  line L161 (-22.4505, -144.9505) -> (-74.9505, -92.4505) construction
  line L162 (-7.43, -137.43) -> (-7.43, -152.57) construction
  line L163 (-7.43, -152.57) -> (-22.57, -152.57) construction
  line L164 (-22.57, -152.57) -> (-22.57, -137.43) construction
  line L165 (-22.57, -137.43) -> (-7.43, -137.43) construction
  line L166 (-25, -152.5) -> (-40.0535, -152.5) construction
  line L167 (-40.0535, -152.5) -> (-40.0535, -145) construction
  line L168 (-40.0535, -145) -> (-25, -145) construction
  line L169 (-25, -145) -> (-25, -152.5) construction
  point P0 (120, 0)
  point P1 (120, -5)
  point P2 (115, -5)
  point P3 (-40, -205)
  point P4 (-40, -210)
  point P5 (-45, -210)
  point P6 (50, -205)
  point P7 (50, -210)
  point P8 (45, -210)
  point P9 (-40, -115)
  point P10 (-40, -120)
  point P11 (-45, -120)
  point P12 (50, -115)
  point P13 (50, -120)
  point P14 (45, -120)
  dimension "d67" = 75
  dimension "d68" = 75
  dimension "d69" = 75
  dimension "d70" = 75
  dimension "d71" = 75
  dimension "d72" = 75
  dimension "d73" = 75
  dimension "d74" = 75
  dimension "d75" = 75
  dimension "d76" = 75
  dimension "d77" = -0.1
  dimension "d78" = -0.1
  dimension "d79" = 0.1
  dimension "d80" = 3
  dimension "d81" = 0.09
  dimension "d82" = -0.09
  dimension "d83" = -0.09
  dimension "d84" = 3
  dimension "d85" = -0.08
  dimension "d86" = -0.08
  dimension "d87" = 0.08
  dimension "d88" = 3
  dimension "d89" = 0.07
  dimension "d90" = 0.07
  dimension "d91" = -0.07
  dimension "d92" = 3
  constraint horizontal L1
  constraint vertical L13
  constraint horizontal L10
  constraint vertical L17
  constraint horizontal L21
  constraint vertical L25
  constraint horizontal L3
  constraint vertical L4
  constraint horizontal L0
  constraint vertical L7
  constraint horizontal L22
  constraint vertical L20
  constraint horizontal L18
  constraint vertical L8
  constraint horizontal L9
  constraint vertical L11
  constraint horizontal L23
  constraint vertical L24
  constraint horizontal L19
  constraint vertical L2
  constraint midpoint L14.start L9
  constraint midpoint L14.end L7
  constraint midpoint L16.start L22
  constraint midpoint L16.end L8
  constraint midpoint L6.start L3
  constraint midpoint L6.end L24
  constraint midpoint L15.start L25
  constraint midpoint L15.end L19
  constraint midpoint L12.start L1
  constraint midpoint L12.end L10
  constraint midpoint L5.start L17
  constraint midpoint L5.end L13
  constraint horizontal L27
  constraint vertical L39
  constraint horizontal L36
  constraint vertical L43
  constraint horizontal L47
  constraint vertical L51
  constraint horizontal L29
  constraint vertical L30
  constraint horizontal L26
  constraint vertical L33
  constraint horizontal L48
  constraint vertical L46
  constraint horizontal L44
  constraint vertical L34
  constraint horizontal L35
  constraint vertical L37
  constraint horizontal L49
  constraint vertical L50
  constraint horizontal L45
  constraint vertical L28
  constraint midpoint L40.start L35
  constraint midpoint L40.end L33
  constraint midpoint L42.start L48
  constraint midpoint L42.end L34
  constraint midpoint L32.start L29
  constraint midpoint L32.end L50
  constraint midpoint L41.start L51
  constraint midpoint L41.end L45
  constraint midpoint L38.start L27
  constraint midpoint L38.end L36
  constraint midpoint L31.start L43
  constraint midpoint L31.end L39
  constraint horizontal L53
  constraint vertical L65
  constraint horizontal L62
  constraint vertical L69
  constraint horizontal L73
  constraint vertical L77
  constraint horizontal L55
  constraint vertical L56
  constraint horizontal L52
  constraint vertical L59
  constraint horizontal L74
  constraint vertical L72
  constraint horizontal L70
  constraint vertical L60
  constraint horizontal L61
  constraint vertical L63
  constraint horizontal L75
  constraint vertical L76
  constraint horizontal L71
  constraint vertical L54
  constraint midpoint L66.start L61
  constraint midpoint L66.end L59
  constraint midpoint L68.start L74
  constraint midpoint L68.end L60
  constraint midpoint L58.start L55
  constraint midpoint L58.end L76
  constraint midpoint L67.start L77
  constraint midpoint L67.end L71
  constraint midpoint L64.start L53
  constraint midpoint L64.end L62
  constraint midpoint L57.start L69
  constraint midpoint L57.end L65
  constraint horizontal L79
  constraint vertical L91
  constraint horizontal L88
  constraint vertical L95
  constraint horizontal L99
  constraint vertical L103
  constraint horizontal L81
  constraint vertical L82
  constraint horizontal L78
  constraint vertical L85
  constraint horizontal L100
  constraint vertical L98
  constraint horizontal L96
  constraint vertical L86
  constraint horizontal L87
  constraint vertical L89
  constraint horizontal L101
  constraint vertical L102
  constraint horizontal L97
  constraint vertical L80
  constraint midpoint L92.start L87
  constraint midpoint L92.end L85
  constraint midpoint L94.start L100
  constraint midpoint L94.end L86
  constraint midpoint L84.start L81
  constraint midpoint L84.end L102
  constraint midpoint L93.start L103
  constraint midpoint L93.end L97
  constraint midpoint L90.start L79
  constraint midpoint L90.end L88
  constraint midpoint L83.start L95
  constraint midpoint L83.end L91
  constraint horizontal L105
  constraint vertical L117
  constraint horizontal L114
  constraint vertical L121
  constraint horizontal L125
  constraint vertical L129
  constraint horizontal L107
  constraint vertical L108
  constraint horizontal L104
  constraint vertical L111
  constraint horizontal L126
  constraint vertical L124
  constraint horizontal L122
  constraint vertical L112
  constraint horizontal L113
  constraint vertical L115
  constraint horizontal L127
  constraint vertical L128
  constraint horizontal L123
  constraint vertical L106
  constraint midpoint L118.start L113
  constraint midpoint L118.end L111
  constraint midpoint L120.start L126
  constraint midpoint L120.end L112
  constraint midpoint L110.start L107
  constraint midpoint L110.end L128
  constraint midpoint L119.start L129
  constraint midpoint L119.end L123
  constraint midpoint L116.start L105
  constraint midpoint L116.end L114
  constraint midpoint L109.start L121
  constraint midpoint L109.end L117
  constraint coincident L36
  constraint coincident L62
  constraint coincident L105
  constraint coincident L79
  measures "d67" distance of L1.start L0.start
  measures "d68" distance of L1.start L10.end
  measures "d69" distance of L27.start L26.start
  measures "d70" distance of L27.start L36.end
  measures "d71" distance of L53.start L52.start
  measures "d72" distance of L53.start L62.end
  measures "d73" distance of L79.start L78.start
  measures "d74" distance of L79.start L88.end
  measures "d75" distance of L105.start L104.start
  measures "d76" distance of L105.start L114.end
ref_plane "Arbeitsebene2" through (-40, 10, 45) normal (0, -1, 0) x (1, 0, 0)